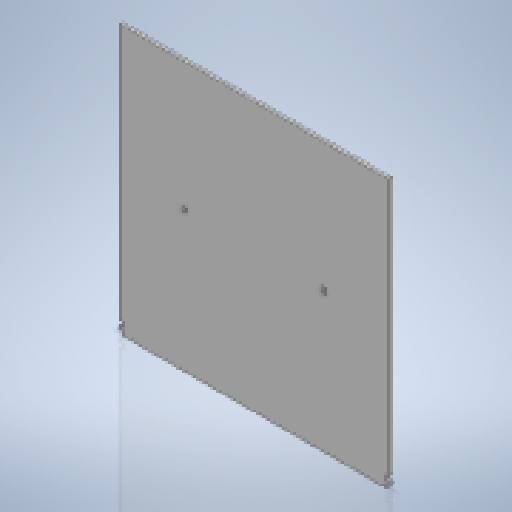
# Autodesk Inventor part: tampa
Saved by Autodesk Inventor 2024.3 (Build 283343000, 343)
## iProperties
Created: 2024-04-25
Part Number: tampa
Material: Genérico
Document SubType Name: Modeling
Designer: joaov
Density: 1 g/cm^3
Appearance: Padrão
Author: joaov
Autodesk Inventor part; units mm, degrees
ref_plane "YZ Plane" through (0, 0, 0) normal (1, 0, 0) x (0, 1, 0)
ref_plane "XZ Plane" through (0, 0, 0) normal (0, 1, 0) x (-1, 0, 0)
ref_plane "XY Plane" through (0, 0, 0) normal (0, 0, 1) x (1, 0, 0)
sketch "Esboço1" plane through (0, 0, 0) normal (0, 0, 1) x (1, 0, 0)
  line L0 (-300, 13) -> (-300, 300)
  line L1 (-300, 300) -> (0, 300)
  line L2 (1, 6) -> (1, 7.5)
  line L3 (1, 6) -> (1, 4.5)
  line L4 (1, 4.5) -> (-3, 4.5)
  line L5 (1, 7.5) -> (-3, 7.5)
  line L6 (-3, 12) -> (-3, 7.5)
  line L7 (-3, 4.5) -> (-3, 0)
  line L8 (-151.5, 0) -> (-151.5, 22.4089)
  line L9 (-297, 0) -> (-3, 0)
  line L10 (-301, 6) -> (-301, 7.5)
  line L11 (-301, 7.5) -> (-297, 7.5)
  line L12 (-301, 6) -> (-301, 4.5)
  line L13 (-301, 4.5) -> (-297, 4.5)
  line L14 (-297, 0) -> (-297, 4.5)
  line L15 (-297, 7.5) -> (-297, 12)
  line L16 (-300, 13) -> (-297, 13)
  line L17 (-297, 13) -> (-297, 12)
  line L18 (-3, 12) -> (-3, 13)
  line L19 (-3, 13) -> (0, 13)
  line L20 (0, 13) -> (0, 300)
  point P0 (0, 0)
  dimension "d2" = 300
  dimension "d14" = 1
  constraints: 42 end point, 10 perpendicular, 5 vertical, 1 horizontal
  measures "d2" distance of L0.end L1.end
  measures "d14" distance of L6.start L18.end
extrude "Extrusão1" add sketch "Esboço1" along normal blind 3
sketch "Esboço2" plane through (0, 0, 3) normal (0, 0, 1) x (1, 0, 0)
  line L0 (-300, 300) -> (-300, 13) projected
  line L1 (0, 13) -> (0, 300) projected
  line L2 (-150, 156.5) -> (-75, 156.5)
  line L3 (-150, 156.5) -> (-225, 156.5)
  line L4 (-225, 156.5) -> (-228, 156.5)
  line L5 (-75, 156.5) -> (-72, 156.5)
  circle A0 centre (-72, 156.5) radius 3
  circle A1 centre (-228, 156.5) radius 3
  point P0 (0, 0)
  dimension "d17" = 75
  dimension "d18" = 75
  dimension "d20" = 3
  dimension "d21" = 3
  constraints: 8 end point, 3 horizontal, 2 coincident, 2 horizontal alignment, 4 other
  measures "d17" distance of L2.start L2.end
  measures "d18" distance of L2.start L3.end
  measures "d20" distance of L3.end L4.end
  measures "d21" distance of L2.end L5.end
extrude "Extrusão2" cut sketch "Esboço2" against normal through all
